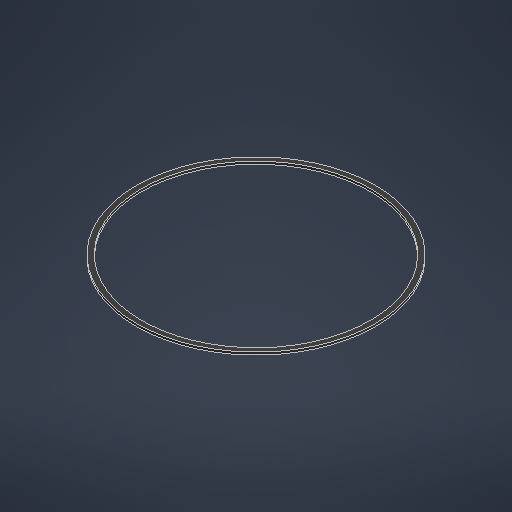
# Autodesk Inventor part: Ring_Dichtung
Saved by Autodesk Inventor 2027 (Build 310192060, 192F)
## iProperties
Created: 2026-08-01
Part Number: Ring_Dichtung
Material: Rubber, Silicone
Document SubType Name: Modeling
Designer: kw
Density: 1.25 g/cm^3
Appearance: Rubber - Black
Author: kw
Autodesk Inventor part; units mm, degrees
ref_plane "YZ Plane" through (0, 0, 0) normal (1, 0, 0) x (0, 1, 0)
ref_plane "XZ Plane" through (0, 0, 0) normal (0, 1, 0) x (-1, 0, 0)
ref_plane "XY Plane" through (0, 0, 0) normal (0, 0, 1) x (1, 0, 0)
sketch "Sketch1" plane through (0, 0, 0) normal (0, 1, 0) x (-1, 0, 0)
  circle A0 centre (0, 0) radius 47
  circle A1 centre (0, 0) radius 42
  circle A2 centre (0, 0) radius 43.5
  circle A3 centre (0, 0) radius 45.5
  dimension "d0" = 94
  dimension "d1" = 84
  dimension "d2" = 87
  dimension "d3" = 91
  constraints: 4 centre point, 4 coincident
  measures "d0" diameter of A0
  measures "d1" diameter of A1
  measures "d2" diameter of A2
  measures "d3" diameter of A3
extrude "Extrusion1" add sketch "Sketch1" along normal blind 1 contours A3
body "Solid1"
